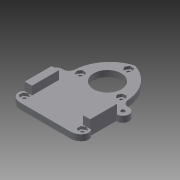
# Autodesk Inventor part: BallBearingHolderBottom
Saved by Autodesk Inventor 2015 (Build 190159000, 159)
## iProperties
Created: 2017-03-08
Part Number: BallBearingHolderBottom
Material: Generic
Document SubType Name: Modeling
Designer: Ernest
Density: 1 g/cm^3
Appearance: Default
Author: Ernest
Autodesk Inventor part; units mm, degrees
ref_plane "YZ Plane" through (0, 0, 0) normal (1, 0, 0) x (0, 1, 0)
ref_plane "XZ Plane" through (0, 0, 0) normal (0, 1, 0) x (-1, 0, 0)
ref_plane "XY Plane" through (0, 0, 0) normal (0, 0, 1) x (1, 0, 0)
sketch "Sketch1" plane through (0, 0, 0) normal (0, 0, 1) x (1, 0, 0)
  circle A0 centre (0, 0) radius 11.5
  line L0 (21.15, -51.53) -> (-21.15, -51.53) construction
  line L1 (-21.15, -51.53) -> (-21.15, -9.23) construction
  line L2 (-21.15, -9.23) -> (21.15, -9.23) construction
  line L3 (21.15, -9.23) -> (21.15, -51.53) construction
  circle A1 centre (0, 17.5) radius 1.6
  circle A2 centre (17, -5.5) radius 1.6
  circle A3 centre (-17, -5.5) radius 1.6
  line L4 (13.6253, -5.9632) -> (14.9115, -2.809)
  line L5 (14.9115, -2.809) -> (18.2862, -2.3458)
  line L6 (18.2862, -2.3458) -> (20.3747, -5.0368)
  line L7 (20.3747, -5.0368) -> (19.0885, -8.191)
  line L8 (19.0885, -8.191) -> (15.7138, -8.6542)
  line L9 (15.7138, -8.6542) -> (13.6253, -5.9632)
  line L10 (-15.7138, -8.6542) -> (-19.0885, -8.191)
  line L11 (-19.0885, -8.191) -> (-20.3747, -5.0368)
  line L12 (-20.3747, -5.0368) -> (-18.2862, -2.3458)
  line L13 (-18.2862, -2.3458) -> (-14.9115, -2.809)
  line L14 (-14.9115, -2.809) -> (-13.6253, -5.9632)
  line L15 (-13.6253, -5.9632) -> (-15.7138, -8.6542)
  line L16 (-1.7032, 14.55) -> (-3.4064, 17.5)
  line L17 (-3.4064, 17.5) -> (-1.7032, 20.45)
  line L18 (-1.7032, 20.45) -> (1.7032, 20.45)
  line L19 (1.7032, 20.45) -> (3.4064, 17.5)
  line L20 (3.4064, 17.5) -> (1.7032, 14.55)
  line L21 (1.7032, 14.55) -> (-1.7032, 14.55)
  line L22 (0, 0) -> (0, 17.5) construction
  line L23 (15.7138, -8.6542) -> (15.7138, -9.23) construction
  line L24 (13.6253, -5.9632) -> (13.1223, -5.6828) construction
  line L25 (21.15, -41.53) -> (27.15, -41.53)
  line L26 (27.15, -41.53) -> (27.15, -19.23)
  line L27 (27.15, -19.23) -> (21.15, -19.23)
  line L28 (21.15, -19.23) -> (21.15, -41.53)
  line L29 (-21.15, -41.53) -> (-27.15, -41.53)
  line L30 (-27.15, -41.53) -> (-27.15, -19.23)
  line L31 (-27.15, -19.23) -> (-21.15, -19.23)
  line L32 (-21.15, -19.23) -> (-21.15, -41.53)
  circle A4 centre (27.75, -14.88) radius 1.6
  circle A5 centre (-27.75, -14.88) radius 1.6
  line L33 (24.8, -16.5832) -> (24.8, -13.1768)
  line L34 (24.8, -13.1768) -> (27.75, -11.4736)
  line L35 (27.75, -11.4736) -> (30.7, -13.1768)
  line L36 (30.7, -13.1768) -> (30.7, -16.5832)
  line L37 (30.7, -16.5832) -> (27.75, -18.2864)
  line L38 (27.75, -18.2864) -> (24.8, -16.5832)
  line L39 (-27.75, -18.2864) -> (-30.7, -16.5832)
  line L40 (-30.7, -16.5832) -> (-30.7, -13.1768)
  line L41 (-30.7, -13.1768) -> (-27.75, -11.4736)
  line L42 (-27.75, -11.4736) -> (-24.8, -13.1768)
  line L43 (-24.8, -13.1768) -> (-24.8, -16.5832)
  line L44 (-24.8, -16.5832) -> (-27.75, -18.2864)
  circle A6 centre (-24.1, -44.9364) radius 1.6
  circle A7 centre (24.1, -44.9364) radius 1.6
  line L45 (-24.1, -48.3427) -> (-27.05, -46.6395)
  line L46 (-27.05, -46.6395) -> (-27.05, -43.2332)
  line L47 (-27.05, -43.2332) -> (-24.1, -41.53)
  line L48 (-24.1, -41.53) -> (-21.15, -43.2332)
  line L49 (-21.15, -43.2332) -> (-21.15, -46.6395)
  line L50 (-21.15, -46.6395) -> (-24.1, -48.3427)
  line L51 (24.1, -48.3427) -> (21.15, -46.6395)
  line L52 (21.15, -46.6395) -> (21.15, -43.2332)
  line L53 (21.15, -43.2332) -> (24.1, -41.53)
  line L54 (24.1, -41.53) -> (27.05, -43.2332)
  line L55 (27.05, -43.2332) -> (27.05, -46.6395)
  line L56 (27.05, -46.6395) -> (24.1, -48.3427)
  arc A8 (-27.3663, -9.8947) -> (-27.15, -19.8439) centre (-27.75, -14.88) ccw
  arc A9 (27.15, -19.8439) -> (27.3663, -9.8947) centre (27.75, -14.88) ccw
  arc A10 (-27.15, -40.9744) -> (-28.2818, -47.6773) centre (-24.1, -44.9364) ccw
  arc A11 (28.2818, -47.6773) -> (27.15, -40.9744) centre (24.1, -44.9364) ccw
  line L57 (21.15, -48.9734) -> (21.15, -51.53)
  line L58 (21.15, -51.53) -> (-21.15, -51.53)
  line L59 (-21.15, -51.53) -> (-21.15, -48.9734)
  arc A12 (1.7467, 22.185) -> (-1.7467, 22.185) centre (0, 17.5) ccw
  arc A13 (-27.3663, -9.8947) -> (-21.9913, -5.2047) centre (-26.9825, -4.9095) ccw
  arc A14 (21.9913, -5.2047) -> (27.3663, -9.8947) centre (26.9825, -4.9095) ccw
  arc A15 (21.15, -51.53) -> (28.2818, -47.6773) centre (21.15, -43.0028) ccw
  arc A16 (-28.2818, -47.6773) -> (-21.15, -51.53) centre (-21.15, -43.0028) ccw
  arc A17 (-1.7467, 22.185) -> (-21.9913, -5.2047) centre (9.1518, -7.047) ccw
  arc A18 (21.9913, -5.2047) -> (1.7467, 22.185) centre (-9.1518, -7.047) ccw
  dimension "d1" = 23
  dimension "d19" = 9.23
  dimension "d20" = 42.3
  dimension "d21" = 21.15
  dimension "d22" = 42.3
  dimension "d23" = 3.2
  dimension "d24" = 3.2
  dimension "d25" = 3.2
  dimension "d26" = 5.5
  dimension "d27" = 17
  dimension "d28" = 5.5
  dimension "d29" = 17
  dimension "d30" = 5.9
  dimension "d31" = 17.5
  dimension "d32" = 5.9
  dimension "d33" = 5.9
  dimension "d35" = 0.5758
  dimension "d36" = 0.5758
  dimension "d37" = 6
  dimension "d38" = 10
  dimension "d39" = 10
  dimension "d40" = 6
  dimension "d41" = 3.2
  dimension "d42" = 3.2
  dimension "d43" = 5.65
  dimension "d44" = 6.6
  dimension "d45" = 6.6
  dimension "d46" = 5.65
  dimension "d47" = 5.9
  dimension "d48" = 5.9
  dimension "d49" = 3.2
  dimension "d50" = 3.2
  dimension "d52" = 2.95
  dimension "d53" = 2.95
  dimension "d54" = 5.9
  dimension "d55" = 5.9
  dimension "d56" = 10
  dimension "d57" = 10
  dimension "d58" = 10
  dimension "d59" = 10
  dimension "d61" = 10
  dimension "d63" = 10
  dimension "d64" = 10
  constraints: 120 end point, 22 point on circle, 19 centre point, 14 coincident, 11 point on line, 10 tangent, 8 parallel, 6 perpendicular, 5 collinear, 3 horizontal, 1 equal length, 1 vertical, 91 other
  measures "d1" diameter of A0
  measures "d19" distance from line of point (0, 0) L2
  measures "d20" distance of L0.start L0.end
  measures "d21" distance from line of point (0, 0) L3
  measures "d22" distance of L2.end L0.start
  measures "d23" diameter of A2
  measures "d24" diameter of A1
  measures "d25" diameter of A3
  measures "d26" vertical distance of A2.centre point (0, 0)
  measures "d27" horizontal distance of point (0, 0) A2.centre
  measures "d28" vertical distance of point (0, 0) A3.centre
  measures "d29" horizontal distance of point (0, 0) A3.centre
  measures "d30" distance between parallel lines of L18 L21
  measures "d31" distance of point (0, 0) A1.centre
  measures "d32" distance between parallel lines of L5 L8
  measures "d33" distance between parallel lines of L13 L10
  measures "d35" distance of L8.end L23.end
  measures "d36" distance from line of L2 L10.start
  measures "d37" distance of L25.start L25.end
  measures "d38" distance between parallel lines of L2 L27
  measures "d39" distance between parallel lines of L25 L0
  measures "d40" distance of L29.start L29.end
  measures "d41" diameter of A5
  measures "d42" diameter of A4
  measures "d43" distance from line of L2 A4.centre
  measures "d44" distance from line of A4.centre L3
  measures "d45" distance from line of L1 A5.centre
  measures "d46" distance from line of L2 A5.centre
  measures "d47" distance between parallel lines of L44 L41
  measures "d48" distance between parallel lines of L34 L37
  measures "d49" diameter of A6
  measures "d50" diameter of A7
  measures "d52" distance from line of L1 A6.centre
  measures "d53" distance from line of L3 A7.centre
  measures "d54" distance between parallel lines of L49 L46
  measures "d55" distance between parallel lines of L55 L52
  measures "d56" diameter of A8
  measures "d57" diameter of A9
  measures "d58" diameter of A10
  measures "d59" diameter of A11
  measures "d61" diameter of A12
  measures "d63" diameter of A13
  measures "d64" diameter of A14
extrude "Extrusion5" add sketch "Sketch1" along normal blind 5 contours L25 L26 A11 A15 L58 A16 A10 L30 L29 L32 L31 A8 A13 A17 A12 A18 A14 A9 L27 L28 | L33 L34 L35 L36 L37 L38 | L39 L40 L41 L42 L43 L44
extrude "Extrusion6" add sketch "Sketch1" along normal blind 12 contours L28 L27 L26 L25 | L30 L31 L32 L29
extrude "Extrusion7" add sketch "Sketch1" along normal blind 2.7 contours L4 L5 L6 L7 L8 L9 | L10 L11 L12 L13 L14 L15 | L16 L17 L18 L19 L20 L21 | L48 L49 L50 L45 L46 L47 | L54 L55 L56 L51 L52 L53
extrude "Extrusion8" cut sketch "Sketch1" along normal blind 3 contours L33 L34 L35 L36 L37 L38 | L39 L40 L41 L42 L43 L44
sketch "Sketch2" plane through (0, 0, 5) normal (0, 0, 1) x (1, 0, 0)
  circle A0 centre (0, 17.5) radius 1.6 projected
  circle A1 centre (-17, -5.5) radius 1.6 projected
  circle A2 centre (-17, -5.5) radius 1.6 projected
  circle A3 centre (-24.1, -44.9364) radius 1.6 projected
  circle A4 centre (24.1, -44.9364) radius 1.6 projected
  circle A5 centre (24.1, -44.9364) radius 1.6 projected
  circle A6 centre (17, -5.5) radius 1.6 projected
  circle A7 centre (17, -5.5) radius 1.6 projected
  circle A8 centre (0, 0) radius 11.5 projected
  circle A9 centre (0, 0) radius 11.5 projected
  dimension "d77" = 23
  dimension "d78" = 17.5
  dimension "d79" = 34
  dimension "d80" = 5.5
  dimension "d81" = 48.2
  dimension "d82" = 44.9364
  measures "d77" diameter of A8
  measures "d78" distance of point (0, 0) A0.centre
  measures "d79" distance of A6.centre A1.centre
  measures "d80" vertical distance of point (0, 0) A1.centre
  measures "d81" distance of A4.centre A3.centre
  measures "d82" vertical distance of point (0, 0) A3.centre
equation "\"d21\" = 0.5 * d20"
equation "\"d22\" = d20"
body "Solid3"
